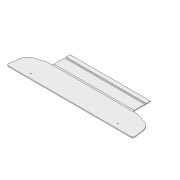
# Autodesk Inventor part: wing
Saved by Autodesk Inventor 2019 (Build 230136000, 136)
## iProperties
Created: 2022-03-25
Part Number: wing
Material: Foam board
Document SubType Name: Modeling
Designer: solyo
Density: 0.096049 g/cm^3
Appearance: Foam
Mass: 61.9295 g
Surface Area: 2852.72 cm^2
Volume: 644.77 cm^3
Author: solyo
Autodesk Inventor part; units mm, degrees
ref_plane "YZ Plane" through (0, 0, 0) normal (1, 0, 0) x (0, 1, 0)
ref_plane "XZ Plane" through (0, 0, 0) normal (0, 1, 0) x (-1, 0, 0)
ref_plane "XY Plane" through (0, 0, 0) normal (0, 0, 1) x (1, 0, 0)
sketch "Sketch1" plane through (0, 0, 0) normal (0, 1, 0) x (-1, 0, 0)
  line L0 (229, 0) -> (-229, 0)
  line L1 (-229, 0) -> (-229, 97)
  line L2 (-229, 97) -> (-241, 97)
  line L3 (-241, 97) -> (-346.9534, 129.9298)
  line L4 (-346.9534, 129.9298) -> (-362, 231)
  line L5 (-362, 231) -> (362, 231)
  line L6 (362, 231) -> (346.9534, 129.9298)
  line L7 (346.9534, 129.9298) -> (241, 97)
  line L8 (229, 0) -> (229, 97)
  line L9 (229, 97) -> (241, 97)
  line L10 (315.7629, 120.236) -> (315.7629, 162.236) construction
  line L11 (315.7629, 162.236) -> (351.7629, 162.236) construction
  arc A0 (315.7629, 120.236) -> (351.7629, 162.236) centre (300.3297, 169.893) ccw construction
  point P0 (0, 0)
  point P1 (0, 0)
  point P2 (0, 231)
  dimension "d0" = 458
  dimension "d2" = 12
  dimension "d3" = 724
  dimension "d5" = 42
  dimension "d6" = 36
  dimension "d8" = 52
  dimension "d30" = 134
  dimension "d37" = 97
  constraints: 24 end point, 3 equal length, 3 perpendicular, 2 horizontal, 2 midpoint, 2 point on circle, 2 point on line, 2 tangent, 2 vertical, 1 centre point, 1 coincident, 1 horizontal alignment, 1 parallel, 1 vertical alignment
  measures "d0" distance of L0.start L0.end
  measures "d2" distance of L8.end L7.end
  measures "d3" distance of L4.end L5.end
  measures "d5" distance of L10.start L10.end
  measures "d6" distance of L10.end L11.end
  measures "d8" radius of A0
  measures "d30" distance between parallel lines of L5 L9
  measures "d37" distance between parallel lines of L0 L9
extrude "Extrusion1" add sketch "Sketch1" along normal blind 5
sketch "Sketch4" plane through (0, 5, 0) normal (0, 1, 0) x (1, 0, 0)
  line L0 (229, 0) -> (-229, 0) projected
  line L1 (-229, 0) -> (-229, -97) projected
  line L2 (-229, -97) -> (-241, -97) projected
  line L3 (-241, -97) -> (-346.9534, -129.9298) projected
  line L4 (-346.9534, -129.9298) -> (-362, -231) projected
  line L5 (-362, -231) -> (362, -231) projected
  line L6 (362, -231) -> (346.9534, -129.9298) projected
  line L7 (346.9534, -129.9298) -> (241, -97) projected
  line L8 (241, -97) -> (229, -97) projected
  line L9 (229, -97) -> (229, 0) projected
  line L10 (-229, -33) -> (229, -33)
  line L11 (-229, -23) -> (229, -23)
  point P0 (0, 0)
  dimension "d39" = 10
  dimension "d40" = 23
  constraints: 4 end point, 4 point on line, 1 horizontal, 1 parallel
  measures "d39" distance between parallel lines of L10 L11
  measures "d40" distance between parallel lines of L0 L11
extrude "Extrusion4" cut sketch "Sketch4" against normal blind 4.5 contours L9 L10 L1 L11
fillet "Fillet2" radius 6 2 edges at (229, 2.5, 97) (-229, 2.5, 97)
fillet "Fillet2" radius 10 2 edges at (-362, 2.5, 231) (362, 2.5, 231)
fillet "Fillet2" radius 52 2 edges at (346.9534, 2.5, 129.9298) (-346.9534, 2.5, 129.9298)
ref_plane "Work Plane1" through (241, 0, 97) normal (0, 0, -1) x (-1, 0, 0)
split body "Split6" result two bodies by plane through (241, 0, 97) normal (0, 0, -1) first body at (76.3333, 0.5, 60.6667)
chamfer "Chamfer2" distance 4.5 angle 45 3 edges at (0, 5, 97) (238, 5, 97) (-238, 5, 97)
sketch "Sketch5" plane through (0, 5, 0) normal (0, 1, 0) x (1, 0, 0)
  line L0 (-249.4011, -202) -> (-247.4011, -202)
  line L1 (-247.4011, -202) -> (-247.4011, -208)
  line L2 (-247.4011, -208) -> (-249.4011, -208)
  line L3 (-249.4011, -208) -> (-249.4011, -202)
  arc A0 (-360.2921, -219.5275) -> (-350.4011, -231) centre (-350.4011, -221) ccw projected
  line L4 (-350.4011, -221) -> (-360.4011, -221) construction
  line L5 (-350.4011, -231) -> (350.4011, -231) construction
  point P0 (0, 0)
  dimension "d46" = 6
  dimension "d47" = 2
  dimension "d48" = 111
  dimension "d49" = 23
  constraints: 10 end point, 2 horizontal, 2 parallel, 1 perpendicular, 1 point on circle
  measures "d46" distance of L2.end L0.start
  measures "d47" distance of L1.end L2.end
  measures "d48" distance from line of L3 L4.end
  measures "d49" distance between parallel lines of L5 L2
extrude "Extrusion5" cut sketch "Sketch5" against normal through all bodies 3
mirror "Mirror1" about plane through (0, 0, 0) normal (1, 0, 0) of "Extrusion5" bodies 3
equation "\"d9\" = Thickness"
equation "\"d41\" = Thickness - Paper"
equation "\"d43\" = Thickness - Paper"
equation "\"Thickness\" = 5"
equation "\"Paper\" = 0.5"
body "Solid13"
body "Solid14"
